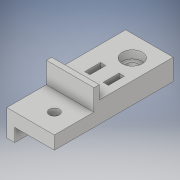
# Autodesk Inventor part: FixedFiber
Saved by Autodesk Inventor 2019 (Build 230136000, 136)
## iProperties
Created: 2019-06-10
Part Number: FixedFiber
Material: Generic
Document SubType Name: Modeling
Designer: aorfi
Density: 1 g/cm^3
Appearance: Default
Author: aorfi
Autodesk Inventor part; units mm, degrees
ref_plane "YZ Plane" through (0, 0, 0) normal (1, 0, 0) x (0, 1, 0)
ref_plane "XZ Plane" through (0, 0, 0) normal (0, 1, 0) x (-1, 0, 0)
ref_plane "XY Plane" through (0, 0, 0) normal (0, 0, 1) x (1, 0, 0)
sketch "Sketch1" plane through (0, 0, 0) normal (0, 1, 0) x (-1, 0, 0)
  line L0 (-7.5, 22.5) -> (10.5, 22.5)
  line L1 (10.5, 22.5) -> (10.5, -22.5)
  line L2 (10.5, -22.5) -> (-7.5, -22.5)
  line L3 (-7.5, -22.5) -> (-7.5, 22.5)
  point P0 (0, 0)
  point P1 (-7.5, 0)
  dimension "d0" = 45
  dimension "d1" = 18
  dimension "d97" = 7.5
  constraints: 8 end point, 2 parallel, 1 horizontal, 1 horizontal alignment, 1 midpoint, 1 perpendicular
  measures "d0" distance of L0.end L1.end
  measures "d1" distance of L1.end L2.end
  measures "d97" distance from line of point (0, 0) L3
extrude "Extrusion1" add sketch "Sketch1" along normal mid plane 8
sketch "Sketch4" plane through (0, 4, 0) normal (0, 1, 0) x (1, 0, 0)
  line L0 (-10.5, -7.5) -> (7.5, -7.5)
  line L1 (7.5, -7.5) -> (7.5, -5.5)
  line L2 (7.5, -5.5) -> (-10.5, -5.5)
  line L3 (-10.5, -5.5) -> (-10.5, -7.5)
  line L4 (-10.5, -22.5) -> (7.5, -22.5) projected
  line L5 (-10.5, 22.5) -> (-10.5, -22.5) projected
  line L6 (7.5, -22.5) -> (7.5, 22.5) projected
  dimension "d57" = 2
  dimension "d58" = 15
  constraints: 8 end point, 2 collinear, 2 parallel, 1 horizontal, 1 perpendicular
  measures "d57" distance of L2.end L0.start
  measures "d58" distance between parallel lines of L4 L0
extrude "Extrusion3" add sketch "Sketch4" along normal blind 5 contours L3 L2 L1 L0
sketch "Sketch5" plane through (0, 4, 0) normal (0, 1, 0) x (1, 0, 0)
  line L0 (-4.5, 7) -> (-2.5, 7)
  line L1 (-2.5, 7) -> (-2.5, 1)
  line L2 (-2.5, 1) -> (-4.5, 1)
  line L3 (-4.5, 1) -> (-4.5, 7)
  line L4 (4.5, 7) -> (2.5, 7)
  line L5 (2.5, 7) -> (2.5, 1)
  line L6 (2.5, 1) -> (4.5, 1)
  line L7 (4.5, 1) -> (4.5, 7)
  line L8 (-3.5, 4) -> (3.5, 4) construction
  line L9 (7.5, -5.5) -> (-7.5, -5.5) construction
  line L10 (-7.5, 7.8654) -> (-7.5, -0.5) construction
  line L11 (-7.5, -0.5) -> (-22.5, -0.5) construction
  line L12 (7.5, -5.5) -> (-10.5, -5.5) projected
  point P0 (0, -5.5)
  point P1 (0, 4)
  point P2 (3.5, 7)
  point P3 (-3.5, 7)
  point P4 (-2.5, 4)
  point P5 (0, 0)
  dimension "d20" = 6
  dimension "d21" = 2
  dimension "d22" = 5
  dimension "d26" = 1.5
  dimension "d31" = 7
  constraints: 24 end point, 5 midpoint, 4 parallel, 4 vertical alignment, 3 horizontal, 3 point on line, 2 collinear, 2 perpendicular
  measures "d20" distance of L2.end L0.start
  measures "d21" distance of L0.start L0.end
  measures "d22" distance between parallel lines of L9 L11
  measures "d26" distance between parallel lines of L2 L11
  measures "d31" distance of L8.start L8.end
extrude "Extrusion4" cut sketch "Sketch5" against normal blind 3
sketch "Sketch7" plane through (-10.5, -4, -12.5) normal (-1, 0, 0) x (0, 0, 1)
  line L0 (20, 8) -> (35, 8) projected
  line L1 (20, 8) -> (35, 8)
  line L2 (35, 8) -> (35, 5)
  line L3 (35, 5) -> (20, 5)
  line L4 (20, 5) -> (20, 8)
  line L5 (35, 8) -> (35, 0) projected
  point P0 (12.5, 4)
  dimension "d59" = 3
  constraints: 8 end point, 2 parallel, 1 collinear, 1 horizontal, 1 perpendicular
  measures "d59" distance between parallel lines of L0 L3
extrude "Extrusion6" cut sketch "Sketch7" against normal through all
sketch "Sketch8" plane through (0, 4, 0) normal (0, 1, 0) x (1, 0, 0)
  line L0 (-10.5, -5.5) -> (-10, -5.5)
  line L1 (-10, -5.5) -> (-10, -3.5)
  line L2 (-10, -3.5) -> (-10.5, -3.5)
  line L3 (-10.5, -3.5) -> (-10.5, -5.5)
  dimension "d60" = 2
  dimension "d61" = 0.5
  constraints: 8 end point, 2 parallel, 1 coincident, 1 horizontal, 1 perpendicular
  measures "d60" distance of L0.end L1.end
  measures "d61" distance of L1.end L2.end
extrude "Extrusion7" add sketch "Sketch8" along normal blind 1
sketch "Sketch13" plane through (-10.5, 1, 22.5) normal (0, 1, 0) x (1, 0, 0)
  line L0 (18, 15) -> (18, 0) projected
  point P0 (10.5, 22.5)
  point P1 (10.5, 7.5)
  point P2 (18, 7.5)
  constraints: 1 horizontal alignment, 1 midpoint, 1 vertical alignment
hole "Hole3" at (0, 1, 15) direction (0, -1, 0) diameter 3.797 end through all clearance for "Flat Head Machine Screw (82)" size "#6" standard "Ansi Unified Screw Threads"
sketch "Sketch12" plane through (0, -4, 0) normal (0, -1, 0) x (1, 0, 0)
  line L0 (7.5, 22.5) -> (-10.5, 22.5) projected
  line L1 (-2.273, 11.063) -> (-4.5461, 15)
  line L2 (-4.5461, 15) -> (-2.273, 18.937)
  line L3 (-2.273, 18.937) -> (2.273, 18.937)
  line L4 (2.273, 18.937) -> (4.5461, 15)
  line L5 (4.5461, 15) -> (2.273, 11.063)
  line L6 (2.273, 11.063) -> (-2.273, 11.063)
  circle A0 centre (0, 15) radius 1.8985 projected
  point P0 (0, 0)
  dimension "d98" = 7.874
  constraints: 12 end point, 1 coincident, 1 horizontal, 13 other
  measures "d98" distance between parallel lines of L6 L3
extrude "Extrusion10" cut sketch "Sketch12" against normal blind 2.7
sketch "Sketch14" plane through (0, 4, 0) normal (0, 1, 0) x (1, 0, 0)
  circle A0 centre (0, 14.5) radius 3.81
  line L0 (7.5, 22.5) -> (-10.5, 22.5) projected
  point P0 (0, 0)
  dimension "d95" = 7.62
  dimension "d96" = 8
  constraints: 1 centre point, 1 vertical alignment
  measures "d95" diameter of A0
  measures "d96" distance from line of L0 A0.centre
extrude "Extrusion11" cut sketch "Sketch14" against normal blind 3
sketch "Sketch15" plane through (0, -4, 0) normal (0, -1, 0) x (1, 0, 0)
  line L0 (-10.5, -22.5) -> (7.5, -22.5) projected
  point P0 (0, 0)
  point P1 (0, -14.5)
  dimension "d87" = 8
  constraints: 1 vertical alignment
  measures "d87" distance from line of L0 point (0, -14.5)
hole "Hole4" at (0, -4, -14.5) direction (0, 1, 0) diameter 4.305 end through all clearance for "Flat Head Machine Screw (82)" size "#6" standard "Ansi Unified Screw Threads"
sketch "Sketch16" plane through (0, -4, 0) normal (0, -1, 0) x (1, 0, 0)
  line L0 (7.5, 22.5) -> (-10.5, 22.5) projected
  line L1 (-10.5, 22.5) -> (-7.5, 22.5)
  line L2 (-7.5, 22.5) -> (-7.5, -22.5)
  line L3 (-7.5, -22.5) -> (-10.5, -22.5)
  line L4 (-10.5, -22.5) -> (-10.5, 22.5)
  line L5 (-10.5, -22.5) -> (7.5, -22.5) projected
  line L6 (7.5, -22.5) -> (7.5, 22.5) projected
  point P0 (0, 0)
  dimension "d102" = 15
  constraints: 8 end point, 2 parallel, 1 collinear, 1 horizontal, 1 perpendicular
  measures "d102" distance between parallel lines of L2 L6
extrude "Extrusion12" add sketch "Sketch16" along normal blind 5 contours L2 L3 L4 L0
body "Solid1"
